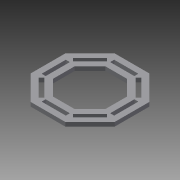
# Autodesk Inventor part: octoBotoTopStemRing
Saved by Autodesk Inventor 2013 (Build 170138000, 138)
## iProperties
Created: 2014-08-27
Part Number: octoBotoTopStemRing
Material: Generic
Document SubType Name: Modeling
Designer: Nano
Density: 1 g/cm^3
Author: Nano
Autodesk Inventor part; units mm, degrees
ref_plane "YZ Plane" through (0, 0, 0) normal (1, 0, 0) x (0, 1, 0)
ref_plane "XZ Plane" through (0, 0, 0) normal (0, 1, 0) x (-1, 0, 0)
ref_plane "XY Plane" through (0, 0, 0) normal (0, 0, 1) x (1, 0, 0)
sketch "Sketch2" plane through (0, 0, 0) normal (0, 1, 0) x (-1, 0, 0)
  line L0 (9.525, -28.575) -> (-9.525, -28.575)
  line L1 (-9.525, -28.575) -> (-9.525, -25.4)
  line L2 (-9.525, -25.4) -> (9.525, -25.4)
  line L3 (9.525, -25.4) -> (9.525, -28.575)
  line L4 (0, -129.3424) -> (0, 132.3553) construction
  line L5 (0, -78.1219) -> (0, -74.9469) construction
  line L6 (26.9408, -13.4704) -> (13.4704, -26.9408)
  line L7 (13.4704, -26.9408) -> (11.2253, -24.6957)
  line L8 (11.2253, -24.6957) -> (24.6957, -11.2253)
  line L9 (24.6957, -11.2253) -> (26.9408, -13.4704)
  line L10 (55.2406, -55.2406) -> (52.9955, -52.9955) construction
  line L11 (28.575, 9.525) -> (28.575, -9.525)
  line L12 (28.575, -9.525) -> (25.4, -9.525)
  line L13 (25.4, -9.525) -> (25.4, 9.525)
  line L14 (25.4, 9.525) -> (28.575, 9.525)
  line L15 (78.1219, 0) -> (74.9469, 0) construction
  line L16 (13.4704, 26.9408) -> (26.9408, 13.4704)
  line L17 (26.9408, 13.4704) -> (24.6957, 11.2253)
  line L18 (24.6957, 11.2253) -> (11.2253, 24.6957)
  line L19 (11.2253, 24.6957) -> (13.4704, 26.9408)
  line L20 (55.2406, 55.2406) -> (52.9955, 52.9955) construction
  line L21 (-9.525, 28.575) -> (9.525, 28.575)
  line L22 (9.525, 28.575) -> (9.525, 25.4)
  line L23 (9.525, 25.4) -> (-9.525, 25.4)
  line L24 (-9.525, 25.4) -> (-9.525, 28.575)
  line L25 (0, 78.1219) -> (0, 74.9469) construction
  line L26 (-26.9408, 13.4704) -> (-13.4704, 26.9408)
  line L27 (-13.4704, 26.9408) -> (-11.2253, 24.6957)
  line L28 (-11.2253, 24.6957) -> (-24.6957, 11.2253)
  line L29 (-24.6957, 11.2253) -> (-26.9408, 13.4704)
  line L30 (-55.2406, 55.2406) -> (-52.9955, 52.9955) construction
  line L31 (-28.575, -9.525) -> (-28.575, 9.525)
  line L32 (-28.575, 9.525) -> (-25.4, 9.525)
  line L33 (-25.4, 9.525) -> (-25.4, -9.525)
  line L34 (-25.4, -9.525) -> (-28.575, -9.525)
  line L35 (-78.1219, 0) -> (-74.9469, 0) construction
  line L36 (-13.4704, -26.9408) -> (-26.9408, -13.4704)
  line L37 (-26.9408, -13.4704) -> (-24.6957, -11.2253)
  line L38 (-24.6957, -11.2253) -> (-11.2253, -24.6957)
  line L39 (-11.2253, -24.6957) -> (-13.4704, -26.9408)
  line L40 (-55.2406, -55.2406) -> (-52.9955, -52.9955) construction
  line L41 (-20.6377, -8.5484) -> (-20.6377, 8.5484)
  line L42 (-20.6377, 8.5484) -> (-8.5484, 20.6377)
  line L43 (-8.5484, 20.6377) -> (8.5484, 20.6377)
  line L44 (8.5484, 20.6377) -> (20.6377, 8.5484)
  line L45 (20.6377, 8.5484) -> (20.6377, -8.5484)
  line L46 (20.6377, -8.5484) -> (8.5484, -20.6377)
  line L47 (8.5484, -20.6377) -> (-8.5484, -20.6377)
  line L48 (-8.5484, -20.6377) -> (-20.6377, -8.5484)
  line L49 (-33.1243, -13.7205) -> (-33.1243, 13.7205)
  line L50 (-33.1243, 13.7205) -> (-13.7205, 33.1243)
  line L51 (-13.7205, 33.1243) -> (13.7205, 33.1243)
  line L52 (13.7205, 33.1243) -> (33.1243, 13.7205)
  line L53 (33.1243, 13.7205) -> (33.1243, -13.7205)
  line L54 (33.1243, -13.7205) -> (13.7205, -33.1243)
  line L55 (13.7205, -33.1243) -> (-13.7205, -33.1243)
  line L56 (-13.7205, -33.1243) -> (-33.1243, -13.7205)
  point P0 (0, 0)
  point P1 (0, 0)
  point P2 (0, 0)
  point P3 (0, 0)
  dimension "d12" = 19.05
  dimension "d13" = 3.175
  dimension "d14" = 9.525
  dimension "d15" = 9.525
  dimension "d18" = 360
  dimension "d20" = 28.575
  constraints: 114 end point, 4 parallel, 2 coincident, 2 horizontal, 1 collinear, 1 perpendicular, 1 vertical, 123 other
  measures "d12" distance of L1.end L2.end
  measures "d13" distance of L0.end L1.end
  measures "d14" distance between parallel lines of L1 L5
  measures "d15" distance between parallel lines of L3 L5
  measures "d20" distance from line of point (0, 0) L0
extrude "Extrusion1" add sketch "Sketch2" along normal blind 3.175
body "Solid1"
